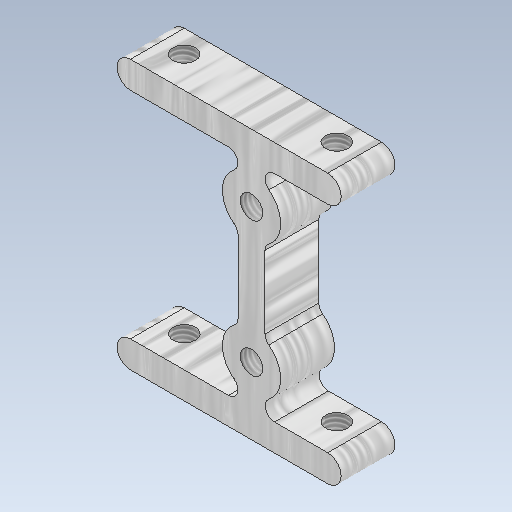
# Autodesk Inventor part: ウィング土台
Saved by Autodesk Inventor 2020.2 (Build 242310000, 310)
## iProperties
Created: 2020-04-12
Part Number: ウィング土台
Material: アルミニウム 7075
Document SubType Name: Modeling
Designer: aoyama
Density: 2.81 g/cm^3
Appearance: サテン - ブラシ仕上げ 重厚
Mass: 3.85654 g
Surface Area: 15.3502 cm^2
Volume: 1.37243 cm^3
Author: aoyama
Autodesk Inventor part; units mm, degrees
ref_plane "YZ Plane" through (0, 0, 0) normal (1, 0, 0) x (0, 1, 0)
ref_plane "XZ Plane" through (0, 0, 0) normal (0, 1, 0) x (-1, 0, 0)
ref_plane "XY Plane" through (0, 0, 0) normal (0, 0, 1) x (1, 0, 0)
sketch "スケッチ1" plane through (0, 0, 0) normal (0, 0, 1) x (1, 0, 0)
  line L0 (0, 0) -> (-25, 0)
  line L1 (-25, 0) -> (-25, 30)
  line L2 (-25, 30) -> (0, 30)
  line L3 (0, 30) -> (0, 0)
  circle A0 centre (-10, 22.5) radius 1.25
  circle A1 centre (-10, 7.5) radius 1.25
  line L4 (-10, 30) -> (-10, 0)
  circle A2 centre (-10, 22.5) radius 3.25
  circle A3 centre (-10, 7.5) radius 3.25
  line L5 (-23.5, 28.5) -> (-1.5, 28.5) construction
  line L6 (-23.5, 27) -> (-1.5, 27)
  line L7 (-1.5, 30) -> (-23.5, 30)
  arc A4 (-23.5, 30) -> (-23.5, 27) centre (-23.5, 28.5) ccw
  arc A5 (-1.5, 27) -> (-1.5, 30) centre (-1.5, 28.5) ccw
  line L8 (-23.5, 1.5) -> (-1.5, 1.5) construction
  line L9 (-23.5, 0) -> (-1.5, 0)
  line L10 (-1.5, 3) -> (-23.5, 3)
  arc A6 (-23.5, 3) -> (-23.5, 0) centre (-23.5, 1.5) ccw
  arc A7 (-1.5, 0) -> (-1.5, 3) centre (-1.5, 1.5) ccw
  line L11 (-10, 28.5) -> (-10, 1.5) construction
  line L12 (-11.5, 28.5) -> (-11.5, 1.5)
  line L13 (-8.5, 1.5) -> (-8.5, 28.5)
  arc A8 (-8.5, 28.5) -> (-11.5, 28.5) centre (-10, 28.5) ccw
  arc A9 (-11.5, 1.5) -> (-8.5, 1.5) centre (-10, 1.5) ccw
  point P0 (-12.5, 28.5)
  point P1 (-12.5, 1.5)
  point P2 (-10, 15)
  point P3 (-11.5, 4.6169)
  point P4 (-11.5, 3)
  point P5 (-1.5, 0)
  point P6 (-8.5, 3)
  point P7 (-8.5, 4.6169)
  point P8 (-8.5, 10.3831)
  point P9 (-8.5, 19.6169)
  point P10 (-8.5, 25.3831)
  point P11 (-8.5, 27)
  point P12 (-11.5, 27)
  point P13 (-11.5, 25.3831)
  point P14 (-11.5, 19.6169)
  point P15 (-11.5, 10.3831)
  dimension "d0" = 25
  dimension "d1" = 30
  dimension "d2" = 2.5
  dimension "d3" = 2.5
  dimension "d4" = 10
  dimension "d5" = 15
  dimension "d6" = 2
  dimension "d7" = 2
  dimension "d8" = 3
  dimension "d9" = 3
  dimension "d10" = 3
  dimension "d11" = 6
  constraints: 34 end point, 16 tangent, 12 point on circle, 10 centre point, 8 point on line, 5 parallel, 3 midpoint, 2 collinear, 1 horizontal, 1 vertical
  measures "d0" distance of L1.end L2.end
  measures "d1" distance of L0.end L1.end
  measures "d2" diameter of A0
  measures "d3" diameter of A1
  measures "d4" distance between parallel lines of L3 L4
  measures "d5" distance of A1.centre A0.centre
  measures "d6" radial gap between concentric circles of A0 A2
  measures "d7" radial gap between concentric circles of A1 A3
  measures "d8" diameter of A5
  measures "d9" diameter of A7
  measures "d10" diameter of A9
  measures "d11" distance from line of A0.centre L5
extrude "押し出し1" add sketch "スケッチ1" along normal blind 6 contours L0 A9 L13 L10 A7 | A9 L12 L10 L4 | L0 A6 L10 L12 A9 | L4 L10 L13 A9 | A5 L6 L13 A8 L2 | L10 L12 A3 L4 | L4 A3 L13 L10 | A3 L12 L4 A1 | L4 A1 A3 L13 | L13 A2 L4 L6 | L6 L4 A8 L13 | A8 L12 L6 A4 L2 | L4 L6 L12 A8 | L13 A3 | A3 L12 | L4 A2 L12 L6 | L13 A2 L4 A0 | A2 L13 | A3 L4 A2 L13 | L12 A2 L4 A3 | L4 A0 A2 L12 | A2 L12
fillet "フィレット1" radius 1.05 12 edges at (-11.5, 25.3831, 3) (-11.5, 27, 3) (-11.5, 19.6169, 3) (-8.5, 27, 3) (-8.5, 25.3831, 3) (-8.5, 19.6169, 3) (-8.5, 10.3831, 3) (-8.5, 4.6169, 3) (-11.5, 4.6169, 3) (-11.5, 10.3831, 3) (-11.5, 3, 3) (-8.5, 3, 3)
thread "ねじ1" size "M3x0.5" class "6H" standard "ANSI Metric M Profile" full length
thread "ねじ2" size "M3x0.5" class "6H" standard "ANSI Metric M Profile" full length
sketch "スケッチ2" plane through (-23.5, 30, 0) normal (0, 1, 0) x (1, 0, 0)
  line L0 (22, 0) -> (0, 0) projected
  line L1 (0, 0) -> (0, -6) projected
  line L2 (22, -6) -> (0, -6) projected
  line L3 (22, 0) -> (22, -6) projected
  circle A0 centre (2.5, -2.5) radius 2.5
  line L4 (22, 0) -> (0, 0) projected
  line L5 (0, 0) -> (0, -6) projected
  circle A1 centre (19.5, -2.5) radius 2.5
  line L6 (22, 0) -> (22, -6) projected
  circle A2 centre (2.5, -2.5) radius 1.25
  circle A3 centre (19.5, -2.5) radius 1.25
  point P0 (23.5, 0)
  dimension "d19" = 5
  dimension "d20" = 5
  dimension "d21" = 2.5
  dimension "d22" = 2.5
  constraints: 4 centre point, 4 tangent, 2 coincident
  measures "d19" diameter of A0
  measures "d20" diameter of A1
  measures "d21" diameter of A2
  measures "d22" diameter of A3
extrude "押し出し2" cut sketch "スケッチ2" against normal blind 30 contours A2 | A3
thread "ねじ3" size "M3x0.5" class "6H" standard "ANSI Metric M Profile" full length
thread "ねじ4" size "M3x0.5" class "6H" standard "ANSI Metric M Profile" full length
thread "ねじ5" size "M3x0.5" class "6H" standard "ANSI Metric M Profile" full length
thread "ねじ6" size "M3x0.5" class "6H" standard "ANSI Metric M Profile" full length
